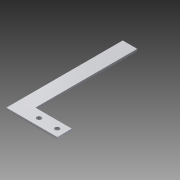
# Autodesk Inventor part: 爪_4
Saved by Autodesk Inventor 2015 (Build 190159000, 159)
## iProperties
Created: 2015-05-18
Part Number: 爪_4
Material: アルミニウム 6061
Document SubType Name: Modeling
Designer: kenta
Density: 2.7 g/cm^3
Appearance: アルミニウム - フラット
Mass: 4.19136 g
Surface Area: 24.4403 cm^2
Volume: 1.55236 cm^3
Author: kenta
Autodesk Inventor part; units mm, degrees
ref_plane "YZ Plane" through (0, 0, 0) normal (1, 0, 0) x (0, 1, 0)
ref_plane "XZ Plane" through (0, 0, 0) normal (0, 1, 0) x (-1, 0, 0)
ref_plane "XY Plane" through (0, 0, 0) normal (0, 0, 1) x (1, 0, 0)
sketch "スケッチ1" plane through (0, 0, 0) normal (0, 0, 1) x (1, 0, 0)
  line L0 (-35, 25) -> (35, 25)
  line L1 (35, 25) -> (35, -25)
  line L2 (35, -25) -> (-35, -25)
  line L3 (-35, -25) -> (-35, 25)
  line L4 (-35, 25) -> (35, -25) construction
  line L5 (35, 25) -> (-35, -25) construction
  point P0 (0, 0)
  dimension "d0" = 70
  dimension "d1" = 50
  constraints: 12 end point, 2 midpoint, 2 parallel, 1 horizontal, 1 perpendicular
  measures "d0" distance of L1.end L2.end
  measures "d1" distance of L0.end L1.end
extrude "押し出し1" add sketch "スケッチ1" along normal blind 1.5
sketch "スケッチ2" plane through (0, 0, 1.5) normal (0, 0, 1) x (1, 0, 0)
  line L0 (-25, 25) -> (25, 25)
  line L1 (25, 25) -> (25, -15)
  line L2 (25, -15) -> (-25, -15)
  line L3 (-25, -15) -> (-25, 25)
  line L4 (-35, 25) -> (-35, -25) projected
  line L5 (35, -25) -> (35, 25) projected
  line L6 (-35, -25) -> (35, -25) projected
  point P0 (0, 0)
  dimension "d4" = 10
  dimension "d5" = 10
  dimension "d6" = 10
  constraints: 8 end point, 2 parallel, 1 horizontal, 1 perpendicular
  measures "d4" distance between parallel lines of L4 L3
  measures "d5" distance between parallel lines of L5 L1
  measures "d6" distance between parallel lines of L6 L2
extrude "押し出し2" cut sketch "スケッチ2" against normal blind 1.5
sketch "スケッチ3" plane through (0, 0, 1.5) normal (0, 0, 1) x (1, 0, 0)
  line L0 (35, -25) -> (35, 25) projected
  line L1 (-35, 25) -> (-35, -25) projected
  line L2 (25, -15) -> (-25, -15) projected
  point P0 (0, 0)
  point P1 (-17.5, -20)
  point P2 (17.5, -20)
  dimension "d9" = 17.5
  dimension "d10" = 17.5
  dimension "d11" = 5
  constraints: 1 horizontal alignment
  measures "d9" distance from line of point (17.5, -20) L0
  measures "d10" distance from line of L1 point (-17.5, -20)
  measures "d11" distance from line of L2 point (17.5, -20)
hole "穴1" at (-17.5, -20, 1.5) at (17.5, -20, 1.5) direction (0, 0, -1) diameter 3.1 end through all
sketch "スケッチ5" plane through (0, 0, 1.5) normal (0, 0, 1) x (1, 0, 0)
  line L0 (-35, -25) -> (35, -25) projected
  line L1 (-35, 25) -> (-35, -25) projected
  point P0 (0, 0)
  point P1 (-5, -20)
  point P2 (5, -20)
  point P3 (-35, 55)
  dimension "d21" = 10
  dimension "d22" = 5
  dimension "d23" = 30
  constraints: 1 horizontal alignment
  measures "d21" distance of point (5, -20) point (-5, -20)
  measures "d22" distance from line of point (5, -20) L0
  measures "d23" distance from line of L1 point (-5, -20)
hole "穴2" at (-5, -20, 1.5) at (5, -20, 1.5) direction (0, 0, -1) diameter 3.1 end through all
sketch "スケッチ6" plane through (0, 0, 1.5) normal (0, 0, 1) x (1, 0, 0)
  line L0 (0, 82.7836) -> (64.7866, 82.7836)
  line L1 (64.7866, 82.7836) -> (64.7866, -43.11)
  line L2 (64.7866, -43.11) -> (0, -43.11)
  line L3 (0, -43.11) -> (0, 82.7836)
  point P0 (0, 0)
  constraints: 8 end point, 2 parallel, 1 horizontal, 1 perpendicular
extrude "押し出し4" cut sketch "スケッチ6" against normal blind 30
sketch "スケッチ7" plane through (-35, 25, 1.5) normal (0, 1, 0) x (1, 0, 0)
  line L0 (0, 0) -> (10, 0)
  line L1 (10, 0) -> (10, 1.5)
  line L2 (10, 1.5) -> (0, 1.5)
  line L3 (0, 1.5) -> (0, 0)
  point P0 (35, 1.5)
  constraints: 8 end point, 2 parallel, 1 horizontal, 1 perpendicular
extrude "押し出し5" add sketch "スケッチ7" along normal blind 30
